Autodesk Fusion 360 part; units mm, degrees
note: some values were not read from the file. Chosen so that the rebuilt part matches the saved one: which face or edge a step refers to. Set by a fixed rule: which sketch regions a step uses.
(part 2 of 2)
sketch "Skizze10" plane through (0, 0, 25) normal (0, 0, 1) x (-1, 0, 0)
  line L0 (-12.516, 9.5118) -> (-14.216, 9.5118)
  line L1 (-14.216, 9.5118) -> (-14.216, 15.5114)
  line L2 (-14.216, 15.5114) -> (-14.516, 15.5114)
  line L3 (-14.516, 15.5114) -> (-14.516, 15.5)
  line L4 (-14.516, 15.5) -> (-15.716, 15.5)
  line L5 (-15.716, 15.5) -> (-15.716, 17.5114)
  line L6 (-15.716, 17.5114) -> (-14.216, 17.5114)
  line L7 (-14.216, 17.5114) -> (-14.216, 23.5233)
  line L8 (-14.216, 23.5233) -> (-15.716, 23.5233)
  line L9 (-15.716, 23.5233) -> (-15.716, 25.5)
  line L10 (-15.716, 25.5) -> (-14.516, 25.5)
  line L11 (-14.516, 25.5) -> (-14.516, 25.5233)
  line L12 (-14.516, 25.5233) -> (-14.216, 25.5233)
  line L13 (-14.216, 25.5233) -> (-14.216, 30.0118)
  line L14 (-14.216, 30.0118) -> (-12.516, 30.0118)
  line L15 (-12.516, 30.0118) -> (-12.516, 32)
  line L16 (-12.516, 32) -> (-20, 32)
  line L17 (-20, 32) -> (-20, 0)
  line L18 (-20, 0) -> (0, 0)
  line L19 (0, 0) -> (0, 32)
  line L20 (0, 32) -> (-4.516, 32)
  line L21 (-4.516, 32) -> (-4.516, 8.1214)
  arc A0 (-12.516, 8.2132) -> (-4.516, 8.1214) centre (-8.5397, 6.1064) ccw
  line L22 (-12.516, 8.2132) -> (-12.516, 9.5118)
  line L23 (-14.216, 14.9954) -> (-15.716, 14.9954)
  line L24 (-15.716, 14.9954) -> (-15.716, 17.9555)
  line L25 (-15.716, 17.9555) -> (-14.216, 17.9555)
  line L26 (-14.216, 17.9555) -> (-14.216, 14.9954)
  line L27 (-14.216, 23.1224) -> (-15.716, 23.1224)
  line L28 (-15.716, 23.1224) -> (-15.716, 25.8589)
  line L29 (-15.716, 25.8589) -> (-14.216, 25.8589)
  line L30 (-14.216, 25.8589) -> (-14.216, 23.1224)
  constraint horizontal L23
  constraint vertical L24
  constraint horizontal L25
  constraint vertical L26
  constraint coincident L1 L23.start
  constraint horizontal L27
  constraint vertical L28
  constraint horizontal L29
  constraint vertical L30
  constraint coincident L7 L27.start
extrude "Extrusion10" [suppressed]
